Pipe bend_v1 (Autodesk Fusion 360 design; units mm, degrees)
Autodesk Fusion 360 part; units mm, degrees
sketch "Esquisse1" plane through (0, 0, 0) normal (0, 0, 1) x (1, 0, 0)
  circle A0 centre (0, 0) radius 12.5
  circle A1 centre (0, 0) radius 15.5
  circle A2 centre (0, 0) radius 18
  dimension "d1" = 25
  dimension "d2" = 31
  dimension "d3" = 36
  constraint coincident A0.centre A1.centre
  constraint concentric A0 A1
  constraint concentric A1 A2
  measures "d1" diameter of A0
  measures "d2" diameter of A1
  measures "d3" diameter of A2
extrude "Extrusion1" add sketch "Esquisse1" along normal blind 28.9 contours A1 | A2
extrude "Extrusion2" add sketch "Esquisse1" against normal blind 13.6 contours A1
sketch "Esquisse2" plane through (0, 0, 28.9) normal (0, 0, 1) x (-1, 0, 0)
  circle A0 centre (0, 0) radius 12.5
  circle A1 centre (0, 0) radius 18
  line L0 (-18, 0) -> (-18, -22)
  constraint coincident A1 L0.start
  constraint tangent A1 L0
  constraint vertical L0
revolve "Révolution1" add sketch "Esquisse2" angle 90 about axis through (18, 0, 28.9) along (0, 1, 0)
sketch "Esquisse3" plane through (18, 0, 0) normal (1, 0, 0) x (0, 1, 0)
  circle A0 centre (0, 46.9) radius 12.5
  circle A1 centre (0, 46.9) radius 18
  circle A2 centre (0, 46.9) radius 15.25
  dimension "d9" = 30.5
  constraint concentric A0 A2
  measures "d9" diameter of A2
extrude "Extrusion3" add sketch "Esquisse3" along normal blind 15 contours A1
equation "d4 = 26.4 mm + 2.5 mm"
